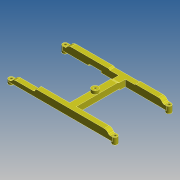
# Autodesk Inventor part: P102
Saved by Autodesk Inventor 2019 (Build 230136000, 136)
## iProperties
Created: 2018-12-18
Part Number: P102
Material: ABS Plastic
Document SubType Name: Modeling
Designer: serge.amoos
Density: 1.06 g/cm^3
Appearance: Canary
Description: Entretoise
Author: serge.amoos
Autodesk Inventor part; units mm, degrees
ref_plane "YZ Plane" through (0, 0, 0) normal (1, 0, 0) x (0, 1, 0)
ref_plane "XZ Plane" through (0, 0, 0) normal (0, 1, 0) x (-1, 0, 0)
ref_plane "XY Plane" through (0, 0, 0) normal (0, 0, 1) x (1, 0, 0)
sketch "Sketch1" plane through (0, 0, 0) normal (0, 0, 1) x (1, 0, 0)
  line L0 (-101.64, 0) -> (83.44, 0) construction
  line L1 (0, -47.332) -> (0, 52.992) construction
  circle A0 centre (-72.2, 35.66) radius 3
  circle A1 centre (-72.2, -30) radius 3
  circle A2 centre (54, -30) radius 3
  circle A3 centre (54, 35.66) radius 3
  line L2 (-72.2, 38.66) -> (54, 38.66)
  line L3 (54, 38.66) -> (54, 32.66)
  line L4 (54, 32.66) -> (-72.2, 32.66)
  line L5 (-72.2, 32.66) -> (-72.2, 38.66)
  line L6 (-72.2, -27) -> (54, -27)
  line L7 (54, -27) -> (54, -33)
  line L8 (54, -33) -> (-72.2, -33)
  line L9 (-72.2, -33) -> (-72.2, -27)
  line L10 (-4, 32.66) -> (4, 32.66)
  line L11 (4, 32.66) -> (4, -27)
  line L12 (4, -27) -> (-4, -27)
  line L13 (-4, -27) -> (-4, 32.66)
  point P0 (0, 0)
  point P1 (0, 32.66)
  dimension "d0" = 6
  dimension "d1" = 6
  dimension "d2" = 6
  dimension "d3" = 6
  dimension "d4" = 54
  dimension "d6" = 30
  dimension "d8" = 8
  dimension "d42" = 65.66
  dimension "d56" = 126.2
  constraints: 24 end point, 6 parallel, 6 vertical alignment, 5 point on line, 3 horizontal, 3 midpoint, 3 perpendicular, 2 horizontal alignment, 8 other
  measures "d4" distance from line of point (54, -30) L1
  measures "d6" distance from line of point (-72.2, -30) L0
  measures "d8" distance between parallel lines of L11 L13
  measures "d42" distance of point (-72.2, -30) point (-72.2, 35.66)
  measures "d56" distance of point (54, -30) point (-72.2, -30)
extrude "Corps" add sketch "Sketch1" along normal blind 9
sketch "Sketch2" plane through (0, 0, 9) normal (0, 0, 1) x (1, 0, 0)
  circle A0 centre (0, 0) radius 4
  dimension "d11" = 8
  constraints: 1 centre point, 1 coincident
  measures "d11" diameter of A0
extrude "Bossage pour vis" add sketch "Sketch2" along normal blind 4
sketch "Sketch3" plane through (0, 0, 13) normal (0, 0, 1) x (1, 0, 0)
  arc A0 (-72.2, 38.66) -> (-72.2, 32.66) centre (-72.2, 35.66) ccw projected
  arc A1 (-72.2, -27) -> (-72.2, -33) centre (-72.2, -30) ccw projected
  arc A2 (54, 32.66) -> (54, 38.66) centre (54, 35.66) ccw projected
  arc A3 (54, -33) -> (54, -27) centre (54, -30) ccw projected
  point P0 (0, 0)
hole "Hole1" at (0, 0, 13) direction (0, 0, -1) diameter 3 depth 8 tip angle 118
sketch "Sketch5" plane through (0, 0, 0) normal (0, 0, -1) x (-1, 0, 0)
  line L0 (-4, 32.66) -> (-54, 32.66) construction
  arc A0 (-54, 38.66) -> (-54, 32.66) centre (-54, 35.66) ccw construction
  line L1 (-54, 38.66) -> (72.2, 38.66) construction
  arc A1 (72.2, 32.66) -> (72.2, 38.66) centre (72.2, 35.66) ccw construction
  line L2 (72.2, 32.66) -> (4, 32.66) construction
  line L3 (4, 32.66) -> (4, -27) construction
  line L4 (4, -27) -> (72.2, -27) construction
  arc A2 (72.2, -33) -> (72.2, -27) centre (72.2, -30) ccw construction
  line L5 (72.2, -33) -> (-54, -33) construction
  arc A3 (-54, -27) -> (-54, -33) centre (-54, -30) ccw construction
  line L6 (-54, -27) -> (-4, -27) construction
  line L7 (-4, -27) -> (-4, 32.66) construction
  circle A4 centre (-54, -30) radius 3
  circle A5 centre (-54, 35.66) radius 3
  circle A6 centre (72.2, -30) radius 3
  circle A7 centre (72.2, 35.66) radius 3
  point P0 (0, 0)
  constraints: 4 coincident, 4 vertical alignment, 8 other
extrude "Pieds" add sketch "Sketch5" along normal blind 3
sketch "Sketch6" plane through (0, 0, 9) normal (0, 0, 1) x (1, 0, 0)
  arc A0 (-72.2, -27) -> (-72.2, -33) centre (-72.2, -30) ccw projected
  line L0 (-72.2, -27) -> (-40.2, -27)
  line L1 (-40.2, -27) -> (-40.2, -33)
  line L2 (-40.2, -33) -> (-72.2, -33)
  point P0 (0, 0)
  dimension "d23" = 32
  constraints: 6 end point, 2 perpendicular, 1 horizontal
  measures "d23" distance from line of L1 A0.centre
extrude "Evidement sur pied 1" cut sketch "Sketch6" against normal blind 3.5
sketch "Sketch7" plane through (0, 0, 5.5) normal (0, 0, 1) x (1, 0, 0)
  arc A0 (-72.2, -27) -> (-72.2, -33) centre (-72.2, -30) ccw projected
  arc A1 (-72.2, -27) -> (-72.2, -33) centre (-72.2, -30) ccw
  line L0 (-72.2, -27) -> (-69.2, -27)
  line L1 (-69.2, -27) -> (-69.2, -33)
  line L2 (-69.2, -33) -> (-72.2, -33)
  point P0 (0, 0)
  dimension "d49" = 3
  constraints: 6 end point, 3 tangent, 2 perpendicular, 2 point on circle, 1 centre point, 1 coincident, 1 horizontal, 1 point on line
  measures "d49" distance from line of L1 A0.centre
extrude "Evidement sur pied 2" cut sketch "Sketch7" against normal blind 3.5
sketch "Sketch8" plane through (-72.2, 38.66, 0) normal (0, 1, 0) x (1, 0, 0)
  line L0 (126.2, 0) -> (0, 0) construction
  line L1 (-3, 3) -> (-3, -9) construction
  line L2 (47, 0) -> (32, 0)
  line L3 (32, 0) -> (32, -2)
  line L4 (32, -2) -> (47, -2)
  line L5 (47, -2) -> (47, 0)
  point P0 (72.2, 0)
  dimension "d29" = 35
  dimension "d30" = 50
  dimension "d31" = 2
  constraints: 8 end point, 2 parallel, 1 horizontal, 1 perpendicular, 1 point on line
  measures "d29" distance between parallel lines of L1 L3
  measures "d30" distance between parallel lines of L1 L5
  measures "d31" distance of L2.end L3.end
extrude "Evidement dessous hor" cut sketch "Sketch8" against normal blind 9
sketch "Sketch9" plane through (54, 35.66, -3) normal (0, 0, -1) x (-1, 0, 0)
  circle A0 centre (0, -65.66) radius 3 projected
  circle A1 centre (126.2, -65.66) radius 3 projected
  circle A2 centre (0, 0) radius 3 projected
  circle A3 centre (126.2, 0) radius 3 projected
  point P0 (54, -35.66)
hole "Hole2" at (-72.2, 35.66, -3) at (-72.2, -30, -3) at (54, -30, -3) at (54, 35.66, -3) direction (0, 0, 1) diameter 3.3 end through all
fillet "Fillet2" radius 2 2 edges at (-40.2, -30, 9) (-40.2, -30, 5.5)
fillet "Fillet5" radius 6 1 edges at (-69.2, -30, 5.5)
fillet "Fillet6" radius 2 1 edges at (-69.2, -30, 2)
sketch "Sketch10" plane through (0, 0, 9) normal (0, 0, 1) x (1, 0, 0)
  line L0 (54, 38.66) -> (-72.2, 38.66) construction
  line L1 (0, 52.992) -> (0, -47.332) construction
  line L2 (-15, 38.66) -> (15, 38.66)
  line L3 (15, 38.66) -> (15, 23.66)
  line L4 (15, 23.66) -> (-15, 23.66)
  line L5 (-15, 23.66) -> (-15, 38.66)
  point P0 (0, 0)
  point P1 (0, 23.66)
  dimension "d43" = 15
  dimension "d44" = 30
  constraints: 8 end point, 2 parallel, 2 point on line, 1 horizontal, 1 midpoint, 1 perpendicular
  measures "d43" distance of L2.end L3.end
  measures "d44" distance of L3.end L4.end
extrude "Evidement dessus" cut sketch "Sketch10" against normal blind 1
fillet "Fillet3" radius 2 2 edges at (0, 23.66, 9) (0, 23.66, 8)
fillet "Fillet4" radius 2 2 edges at (-15, 35.66, 9) (15, 35.66, 9)
sketch "Sketch11" plane through (0, 0, 0) normal (0, 0, -1) x (-1, 0, 0)
  line L0 (-4, -27) -> (-4, 32.66) construction
  line L1 (4, 32.66) -> (4, -27) construction
  line L2 (-54, 38.66) -> (25.2, 38.66) construction
  line L3 (-4, 25.66) -> (4, 25.66)
  line L4 (4, 25.66) -> (4, -20)
  line L5 (4, -20) -> (-4, -20)
  line L6 (-4, -20) -> (-4, 25.66)
  line L7 (38.2, -33) -> (-54, -33) projected
  point P0 (0, 0)
  dimension "d52" = 13
  dimension "d57" = 13
  constraints: 8 end point, 2 parallel, 2 point on line, 1 horizontal, 1 perpendicular
  measures "d52" distance between parallel lines of L3 L2
  measures "d57" distance between parallel lines of L7 L5
extrude "Evidement dessous 2" cut sketch "Sketch11" against normal blind 1.5
sketch "Sketch12" plane through (0, 0, 9) normal (0, 0, 1) x (1, 0, 0)
  line L0 (49, 44.7152) -> (65.9064, 44.7152)
  line L1 (65.9064, 44.7152) -> (65.9064, -37.1821)
  line L2 (65.9064, -37.1821) -> (49, -37.1821)
  line L3 (49, -37.1821) -> (49, 44.7152)
  line L4 (-77.8885, 44.7152) -> (-67.2, 44.7152)
  line L5 (-67.2, 44.7152) -> (-67.2, 25.3936)
  line L6 (-67.2, 25.3936) -> (-77.8885, 25.3936)
  line L7 (-77.8885, 25.3936) -> (-77.8885, 44.7152)
  circle A0 centre (-72.2, 35.66) radius 1.65 projected
  circle A1 centre (54, 35.66) radius 1.65 projected
  point P0 (0, 0)
  dimension "d58" = 5
  dimension "d59" = 5
  constraints: 16 end point, 4 parallel, 2 horizontal, 2 perpendicular, 1 point on line
  measures "d58" distance from line of L5 A0.centre
  measures "d59" distance from line of L3 A1.centre
extrude "Extrusion9" cut sketch "Sketch12" against normal blind 4
fillet "Fillet7" radius 2 3 edges at (49, 35.66, 5) (49, -30, 5) (-67.2, 35.66, 5)
fillet "Fillet8" radius 6 3 edges at (49, 35.66, 9) (49, -30, 9) (-67.2, 35.66, 9)
equation "\"d1\" = d0"
equation "\"d2\" = d0"
equation "\"d3\" = d0"
equation "\"d57\" = d52"
equation "\"d59\" = d58"
body "Solid1"
